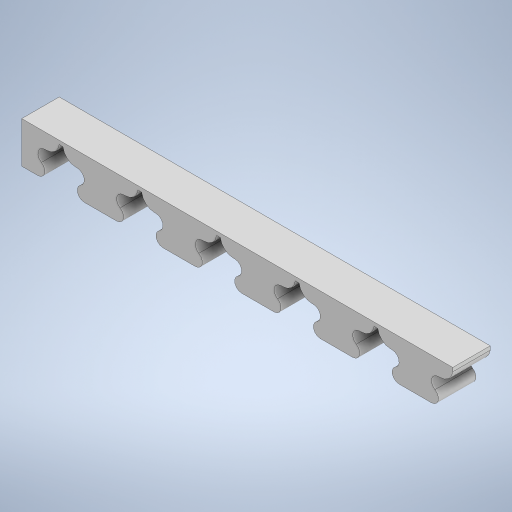
# Autodesk Inventor part: Zipperteethv3
Saved by Autodesk Inventor 2023.1 (Build 271208000, 208)
## iProperties
Created: 2022-10-04
Part Number: Zipperteethv3
Material: Generic
Document SubType Name: Modeling
Designer: Grimm
Density: 1 g/cm^3
Appearance: Default
Author: Grimm
Autodesk Inventor part; units mm, degrees
ref_plane "YZ Plane" through (0, 0, 0) normal (1, 0, 0) x (0, 1, 0)
ref_plane "XZ Plane" through (0, 0, 0) normal (0, 1, 0) x (-1, 0, 0)
ref_plane "XY Plane" through (0, 0, 0) normal (0, 0, 1) x (1, 0, 0)
sketch "Sketch1" plane through (0, 0, 0) normal (0, 0, 1) x (1, 0, 0)
  line L0 (0, 0) -> (21, 0)
  line L1 (21, 0) -> (21, 11)
  line L2 (21, 11) -> (0, 11)
  line L3 (0, 11) -> (0, 0)
  dimension "d0" = 21
  dimension "d1" = 11
  constraints: 8 end point, 2 parallel, 1 horizontal, 1 perpendicular
  measures "d0" distance of L2.end L1.end
  measures "d1" distance of L0.end L1.end
extrude "Extrusion1" add sketch "Sketch1" along normal blind 10
sketch "Sketch2" plane through (0, 0, 10) normal (0, 0, 1) x (1, 0, 0)
  line L0 (0, 0) -> (21, 0) projected
  arc A0 (4.3181, 0) -> (5.25, 3.5) centre (4.3181, 1.8741) ccw
  arc A1 (6.1819, 7) -> (5.25, 3.5) centre (6.1819, 5.1259) ccw
  arc A2 (15.75, 3.5) -> (16.6819, 0) centre (16.6819, 1.8741) ccw
  arc A3 (15.75, 3.5) -> (14.8181, 7) centre (14.8181, 5.1259) ccw
  line L1 (6.1819, 7) -> (14.8181, 7)
  line L2 (21, 11) -> (0, 11) projected
  line L3 (4.3181, 1.8741) -> (6.1819, 5.1259) construction
  line L4 (16.6819, 1.8741) -> (14.8181, 5.1259) construction
  line L5 (0, 11) -> (0, 0) construction
  line L6 (21, 0) -> (21, 11) construction
  point P0 (10.5, 7)
  point P1 (15.75, 3.5)
  dimension "d7" = 10.5
  dimension "d9" = 7
  dimension "d13" = 10.5
  constraints: 8 point on circle, 6 end point, 6 tangent, 4 centre point, 3 equal radius, 3 midpoint, 2 point on line, 1 horizontal
  measures "d7" distance of A2.start A0.end
  measures "d9" distance between parallel lines of L0 L1
  measures "d13" distance from line of L5 point (10.5, 7)
extrude "Extrusion2" cut sketch "Sketch2" against normal through all
sketch "Sketch3" plane through (0, 0, 10) normal (0, 0, 1) x (1, 0, 0)
  line L0 (21, 11) -> (0, 11) projected
  line L1 (14.8181, 7) -> (6.1819, 7) projected
  arc A0 (6.6147, 7) -> (10, 10) centre (6.6147, 10.41) ccw
  arc A1 (11, 10) -> (14.3853, 7) centre (14.3853, 10.41) ccw
  line L2 (10, 10) -> (11, 10)
  line L3 (6.1819, 7) -> (14.8181, 7) projected
  line L4 (10.5, 10) -> (10.5, 11) construction
  point P0 (0, 0)
  dimension "d15" = 1
  dimension "d16" = 1
  constraints: 4 end point, 4 point on circle, 2 centre point, 2 midpoint, 2 point on line, 2 tangent, 1 equal radius, 1 vertical
  measures "d15" distance of L2.start L2.end
  measures "d16" distance between parallel lines of L0 L2
extrude "Extrusion3" cut sketch "Sketch3" against normal through all
pattern_linear "Rectangular Pattern1" count 6 spacing 21 along (1, 0, 0)
sketch "Sketch4" plane through (0, 0, 10) normal (0, 0, 1) x (1, 0, 0)
  line L0 (115, 10) -> (116, 10) projected
  line L1 (115, 10) -> (115, 11)
  line L2 (126, 11) -> (0, 11) projected
  line L3 (121.6819, 0) -> (126, 0) projected
  line L4 (121.6819, 0) -> (126, 0)
  line L5 (126, 0) -> (126, 11)
  line L6 (126, 0) -> (126, 11) projected
  line L7 (126, 11) -> (115, 11)
  arc A0 (116, 10) -> (119.3853, 7) centre (119.3853, 10.41) ccw projected
  line L8 (115, 10) -> (116, 10)
  line L9 (119.3853, 7) -> (119.8181, 7) projected
  arc A1 (116, 10) -> (119.3853, 7) centre (119.3853, 10.41) ccw
  arc A2 (120.75, 3.5) -> (119.8181, 7) centre (119.8181, 5.1259) ccw projected
  line L10 (119.3853, 7) -> (119.8181, 7)
  arc A3 (120.75, 3.5) -> (119.8181, 7) centre (119.8181, 5.1259) ccw
  arc A4 (120.75, 3.5) -> (121.6819, 0) centre (121.6819, 1.8741) ccw projected
  arc A5 (120.75, 3.5) -> (121.6819, 0) centre (121.6819, 1.8741) ccw
  point P0 (0, 0)
  constraints: 12 end point, 7 point on circle, 5 tangent, 3 centre point, 3 horizontal, 2 perpendicular, 1 point on line, 1 vertical
extrude "Extrusion4" cut sketch "Sketch4" against normal through all
body "Solid1"
